Autodesk Fusion 360 part; units mm, degrees
(part 2 of 2)
sketch "스케치2 (4)" plane through (0, 0, 0) normal (0, 0, 1) x (1, 0, 0) in component "right-switch"
  line L0 (143.11, 0) -> (143.11, 105.25)
  line L1 (163.11, 0) -> (338.56, 0)
  line L2 (338.56, 0) -> (338.56, 105.25)
  line L3 (338.56, 105.25) -> (163.11, 105.25)
  line L4 (163.11, 105.25) -> (163.11, 0)
  line L5 (143.11, 105.25) -> (0, 105.25)
  line L6 (322.035, 21.525) -> (336.035, 21.525)
  line L7 (336.035, 21.525) -> (336.035, 7.525)
  line L8 (336.035, 7.525) -> (322.035, 7.525)
  line L9 (322.035, 7.525) -> (322.035, 21.525)
  line L10 (302.985, 21.525) -> (316.985, 21.525)
  line L11 (302.985, 7.525) -> (302.985, 21.525)
  line L12 (316.985, 21.525) -> (316.985, 7.525)
  line L13 (316.985, 7.525) -> (302.985, 7.525)
  line L14 (283.935, 21.525) -> (297.935, 21.525)
  line L15 (283.935, 7.525) -> (283.935, 21.525)
  line L16 (297.935, 21.525) -> (297.935, 7.525)
  line L17 (297.935, 7.525) -> (283.935, 7.525)
  line L18 (264.885, 21.525) -> (278.885, 21.525)
  line L19 (264.885, 7.525) -> (264.885, 21.525)
  line L20 (278.885, 21.525) -> (278.885, 7.525)
  line L21 (278.885, 7.525) -> (264.885, 7.525)
  line L22 (245.835, 21.525) -> (259.835, 21.525)
  line L23 (245.835, 7.525) -> (245.835, 21.525)
  line L24 (259.835, 21.525) -> (259.835, 7.525)
  line L25 (259.835, 7.525) -> (245.835, 7.525)
  line L26 (324.1287, 59.625) -> (324.1287, 53.625)
  line L27 (324.1287, 53.625) -> (325.6287, 53.625)
  line L28 (325.6287, 58.125) -> (332.4287, 58.125)
  line L29 (308.6287, 47.125) -> (301.8287, 47.125)
  line L30 (324.1287, 51.625) -> (324.1287, 45.625)
  line L31 (301.8287, 47.125) -> (301.8287, 58.125)
  line L32 (308.6287, 58.125) -> (308.6287, 53.625)
  line L33 (301.8287, 58.125) -> (308.6287, 58.125)
  line L34 (308.6287, 53.625) -> (310.1287, 53.625)
  line L35 (308.6287, 51.625) -> (308.6287, 47.125)
  line L36 (310.1287, 51.625) -> (308.6287, 51.625)
  line L37 (310.1287, 59.625) -> (324.1287, 59.625)
  line L38 (310.1287, 45.625) -> (310.1287, 51.625)
  line L39 (310.1287, 53.625) -> (310.1287, 59.625)
  line L40 (325.6287, 53.625) -> (325.6287, 58.125)
  line L41 (324.1287, 45.625) -> (310.1287, 45.625)
  line L42 (332.4287, 47.125) -> (325.6287, 47.125)
  line L43 (325.6287, 47.125) -> (325.6287, 51.625)
  line L44 (332.4287, 58.125) -> (332.4287, 47.125)
  line L45 (325.6287, 51.625) -> (324.1287, 51.625)
  line L46 (322.035, 40.575) -> (336.035, 40.575)
  line L47 (336.035, 40.575) -> (336.035, 26.575)
  line L48 (336.035, 26.575) -> (322.035, 26.575)
  line L49 (322.035, 26.575) -> (322.035, 40.575)
  line L50 (312.3662, 26.575) -> (298.3662, 26.575)
  line L51 (312.3662, 40.575) -> (312.3662, 26.575)
  line L52 (298.3663, 40.575) -> (312.3663, 40.575)
  line L53 (298.3663, 26.575) -> (298.3663, 40.575)
  line L54 (288.6975, 26.575) -> (274.6975, 26.575)
  line L55 (288.6975, 40.575) -> (288.6975, 26.575)
  line L56 (274.6975, 40.575) -> (288.6975, 40.575)
  line L57 (274.6975, 26.575) -> (274.6975, 40.575)
  line L58 (255.6475, 40.575) -> (269.6475, 40.575)
  line L59 (255.6475, 26.575) -> (255.6475, 40.575)
  line L60 (269.6475, 40.575) -> (269.6475, 26.575)
  line L61 (269.6475, 26.575) -> (255.6475, 26.575)
  line L62 (236.5975, 40.575) -> (250.5975, 40.575)
  line L63 (236.5975, 26.575) -> (236.5975, 40.575)
  line L64 (250.5975, 40.575) -> (250.5975, 26.575)
  line L65 (250.5975, 26.575) -> (236.5975, 26.575)
  line L66 (217.5475, 40.575) -> (231.5475, 40.575)
  line L67 (217.5475, 26.575) -> (217.5475, 40.575)
  line L68 (231.5475, 40.575) -> (231.5475, 26.575)
  line L69 (231.5475, 26.575) -> (217.5475, 26.575)
  line L70 (198.4975, 40.575) -> (212.4975, 40.575)
  line L71 (198.4975, 26.575) -> (198.4975, 40.575)
  line L72 (212.4975, 40.575) -> (212.4975, 26.575)
  line L73 (212.4975, 26.575) -> (198.4975, 26.575)
  line L74 (179.4475, 40.575) -> (193.4475, 40.575)
  line L75 (179.4475, 26.575) -> (179.4475, 40.575)
  line L76 (193.4475, 40.575) -> (193.4475, 26.575)
  line L77 (193.4475, 26.575) -> (179.4475, 26.575)
  line L78 (193.4475, 7.525) -> (179.4475, 7.525)
  line L79 (193.4475, 21.525) -> (193.4475, 7.525)
  line L80 (179.4475, 7.525) -> (179.4475, 21.525)
  line L81 (179.4475, 21.525) -> (193.4475, 21.525)
  line L82 (212.6412, 15.525) -> (212.6412, 21.525)
  line L83 (228.1412, 15.525) -> (228.1412, 20.025)
  line L84 (228.1412, 9.025) -> (228.1412, 13.525)
  line L85 (204.3412, 20.025) -> (211.1412, 20.025)
  line L86 (204.3412, 9.025) -> (204.3412, 20.025)
  line L87 (228.1412, 20.025) -> (234.9412, 20.025)
  line L88 (226.6412, 7.525) -> (212.6412, 7.525)
  line L89 (211.1412, 15.525) -> (212.6412, 15.525)
  line L90 (211.1412, 9.025) -> (204.3412, 9.025)
  line L91 (212.6412, 13.525) -> (211.1412, 13.525)
  line L92 (211.1412, 20.025) -> (211.1412, 15.525)
  line L93 (211.1412, 13.525) -> (211.1412, 9.025)
  line L94 (226.6412, 13.525) -> (226.6412, 7.525)
  line L95 (234.9412, 20.025) -> (234.9412, 9.025)
  line L96 (212.6412, 21.525) -> (226.6412, 21.525)
  line L97 (226.6412, 21.525) -> (226.6412, 15.525)
  line L98 (226.6412, 15.525) -> (228.1412, 15.525)
  line L99 (212.6412, 7.525) -> (212.6412, 13.525)
  line L100 (234.9412, 9.025) -> (228.1412, 9.025)
  line L101 (228.1412, 13.525) -> (226.6412, 13.525)
  line L102 (281.6975, 45.625) -> (281.6975, 59.625)
  line L103 (295.6975, 59.625) -> (295.6975, 45.625)
  line L104 (281.6975, 59.625) -> (295.6975, 59.625)
  line L105 (295.6975, 45.625) -> (281.6975, 45.625)
  line L106 (262.6475, 59.625) -> (276.6475, 59.625)
  line L107 (276.6475, 59.625) -> (276.6475, 45.625)
  line L108 (276.6475, 45.625) -> (262.6475, 45.625)
  line L109 (262.6475, 45.625) -> (262.6475, 59.625)
  line L110 (243.5975, 59.625) -> (257.5975, 59.625)
  line L111 (257.5975, 59.625) -> (257.5975, 45.625)
  line L112 (257.5975, 45.625) -> (243.5975, 45.625)
  line L113 (243.5975, 45.625) -> (243.5975, 59.625)
  line L114 (224.5475, 59.625) -> (238.5475, 59.625)
  line L115 (238.5475, 59.625) -> (238.5475, 45.625)
  line L116 (238.5475, 45.625) -> (224.5475, 45.625)
  line L117 (224.5475, 45.625) -> (224.5475, 59.625)
  line L118 (205.4975, 59.625) -> (219.4975, 59.625)
  line L119 (219.4975, 59.625) -> (219.4975, 45.625)
  line L120 (219.4975, 45.625) -> (205.4975, 45.625)
  line L121 (205.4975, 45.625) -> (205.4975, 59.625)
  line L122 (186.4475, 59.625) -> (200.4475, 59.625)
  line L123 (200.4475, 59.625) -> (200.4475, 45.625)
  line L124 (200.4475, 45.625) -> (186.4475, 45.625)
  line L125 (186.4475, 45.625) -> (186.4475, 59.625)
  line L126 (331.2725, 64.675) -> (317.2725, 64.675)
  line L127 (317.2725, 78.675) -> (331.2725, 78.675)
  line L128 (317.2725, 64.675) -> (317.2725, 78.675)
  line L129 (331.2725, 78.675) -> (331.2725, 64.675)
  line L130 (309.985, 64.675) -> (295.985, 64.675)
  line L131 (309.985, 78.675) -> (309.985, 64.675)
  line L132 (295.985, 78.675) -> (309.985, 78.675)
  line L133 (295.985, 64.675) -> (295.985, 78.675)
  line L134 (290.935, 78.675) -> (290.935, 64.675)
  line L135 (276.935, 78.675) -> (290.935, 78.675)
  line L136 (290.935, 64.675) -> (276.935, 64.675)
  line L137 (276.935, 64.675) -> (276.935, 78.675)
  line L138 (271.885, 78.675) -> (271.885, 64.675)
  line L139 (257.885, 78.675) -> (271.885, 78.675)
  line L140 (271.885, 64.675) -> (257.885, 64.675)
  line L141 (257.885, 64.675) -> (257.885, 78.675)
  line L142 (252.835, 78.675) -> (252.835, 64.675)
  line L143 (238.835, 78.675) -> (252.835, 78.675)
  line L144 (252.835, 64.675) -> (238.835, 64.675)
  line L145 (238.835, 64.675) -> (238.835, 78.675)
  line L146 (233.785, 78.675) -> (233.785, 64.675)
  line L147 (219.785, 78.675) -> (233.785, 78.675)
  line L148 (233.785, 64.675) -> (219.785, 64.675)
  line L149 (219.785, 64.675) -> (219.785, 78.675)
  line L150 (214.735, 78.675) -> (214.735, 64.675)
  line L151 (200.735, 78.675) -> (214.735, 78.675)
  line L152 (214.735, 64.675) -> (200.735, 64.675)
  line L153 (200.735, 64.675) -> (200.735, 78.675)
  line L154 (195.685, 78.675) -> (195.685, 64.675)
  line L155 (181.685, 78.675) -> (195.685, 78.675)
  line L156 (195.685, 64.675) -> (181.685, 64.675)
  line L157 (181.685, 64.675) -> (181.685, 78.675)
  line L158 (328.01, 85.225) -> (328.01, 89.725)
  line L159 (328.01, 89.725) -> (326.51, 89.725)
  line L160 (312.51, 89.725) -> (311.01, 89.725)
  line L161 (328.01, 91.725) -> (328.01, 96.225)
  line L162 (326.51, 83.725) -> (312.51, 83.725)
  line L163 (312.51, 83.725) -> (312.51, 89.725)
  line L164 (311.01, 96.225) -> (311.01, 91.725)
  line L165 (312.51, 97.725) -> (326.51, 97.725)
  line L166 (326.51, 97.725) -> (326.51, 91.725)
  line L167 (326.51, 91.725) -> (328.01, 91.725)
  line L168 (326.51, 89.725) -> (326.51, 83.725)
  line L169 (304.21, 85.225) -> (304.21, 96.225)
  line L170 (311.01, 91.725) -> (312.51, 91.725)
  line L171 (304.21, 96.225) -> (311.01, 96.225)
  line L172 (334.81, 96.225) -> (334.81, 85.225)
  line L173 (311.01, 89.725) -> (311.01, 85.225)
  line L174 (312.51, 91.725) -> (312.51, 97.725)
  line L175 (334.81, 85.225) -> (328.01, 85.225)
  line L176 (328.01, 96.225) -> (334.81, 96.225)
  line L177 (311.01, 85.225) -> (304.21, 85.225)
  line L178 (286.46, 97.725) -> (300.46, 97.725)
  line L179 (300.46, 97.725) -> (300.46, 83.725)
  line L180 (300.46, 83.725) -> (286.46, 83.725)
  line L181 (286.46, 83.725) -> (286.46, 97.725)
  line L182 (281.41, 83.725) -> (267.41, 83.725)
  line L183 (281.41, 97.725) -> (281.41, 83.725)
  line L184 (267.41, 97.725) -> (281.41, 97.725)
  line L185 (267.41, 83.725) -> (267.41, 97.725)
  line L186 (262.36, 83.725) -> (248.36, 83.725)
  line L187 (262.36, 97.725) -> (262.36, 83.725)
  line L188 (248.36, 97.725) -> (262.36, 97.725)
  line L189 (248.36, 83.725) -> (248.36, 97.725)
  line L190 (243.31, 83.725) -> (229.31, 83.725)
  line L191 (243.31, 97.725) -> (243.31, 83.725)
  line L192 (229.31, 97.725) -> (243.31, 97.725)
  line L193 (229.31, 83.725) -> (229.31, 97.725)
  line L194 (224.26, 83.725) -> (210.26, 83.725)
  line L195 (224.26, 97.725) -> (224.26, 83.725)
  line L196 (210.26, 97.725) -> (224.26, 97.725)
  line L197 (210.26, 83.725) -> (210.26, 97.725)
  line L198 (205.21, 83.725) -> (191.21, 83.725)
  line L199 (205.21, 97.725) -> (205.21, 83.725)
  line L200 (191.21, 97.725) -> (205.21, 97.725)
  line L201 (191.21, 83.725) -> (191.21, 97.725)
  line L202 (186.16, 83.725) -> (172.16, 83.725)
  line L203 (186.16, 97.725) -> (186.16, 83.725)
  line L204 (172.16, 97.725) -> (186.16, 97.725)
  line L205 (172.16, 83.725) -> (172.16, 97.725)
  circle A0 centre (167.11, 101.25) radius 1.55
  circle A1 centre (167.11, 4) radius 1.5
  circle A2 centre (167.11, 4) radius 1.55
  circle A3 centre (266.36, 4) radius 1.55
  circle A4 centre (258.36, 4) radius 1.55
  circle A5 centre (334.56, 4) radius 1.55
  circle A6 centre (334.56, 101.25) radius 1.55
  circle A7 centre (266.36, 101.25) radius 1.55
  circle A8 centre (258.36, 101.25) radius 1.55
  point P0 (143.11, 105.25)
  point P1 (143.11, 0)
  dimension "d237" = 20
  dimension "d238" = 175.45
  dimension "d239" = 14
  dimension "d240" = 14
  dimension "d241" = 7.525
  dimension "d242" = 2.525
  dimension "d246" = 0
  dimension "d251" = 14
  dimension "d252" = 14
  dimension "d253" = 6.8
  dimension "d254" = 11
  dimension "d255" = 1.5
  dimension "d256" = 4.5
  dimension "d257" = 6
  dimension "d261" = 14
  dimension "d262" = 14
  dimension "d263" = 19.05
  dimension "d264" = 2.525
  dimension "d265" = 14
  dimension "d266" = 14
  dimension "d267" = 9.6687
  dimension "d268" = 14
  dimension "d269" = 14
  dimension "d270" = 9.6688
  dimension "d274" = 0
  dimension "d275" = 14
  dimension "d276" = 14
  dimension "d277" = 6.8
  dimension "d278" = 11
  dimension "d279" = 1.5
  dimension "d280" = 4.5
  dimension "d281" = 6
  dimension "d282" = 19.1937
  dimension "d283" = 19.05
  dimension "d284" = 14.4313
  dimension "d285" = 14
  dimension "d286" = 14
  dimension "d287" = 14.4313
  dimension "d291" = 0
  dimension "d292" = 14
  dimension "d293" = 14
  dimension "d294" = 19.05
  dimension "d295" = 7.2875
  dimension "d296" = 14
  dimension "d297" = 14
  dimension "d298" = 7.2875
  dimension "d302" = 0
  dimension "d303" = 14
  dimension "d304" = 14
  dimension "d305" = 6.8
  dimension "d306" = 11
  dimension "d307" = 1.5
  dimension "d308" = 4.5
  dimension "d309" = 6
  dimension "d310" = 19.05
  dimension "d311" = 12.05
  dimension "d312" = 14
  dimension "d313" = 14
  dimension "d314" = 12.05
  dimension "d318" = 0
  dimension "d319" = 3.1
  dimension "d320" = 4
  dimension "d321" = 4
  dimension "d322" = 3
  dimension "d323" = 4
  dimension "d324" = 4
  dimension "d325" = 3.1
  dimension "d326" = 3.1
  dimension "d327" = 72.2
  dimension "d328" = 4
  dimension "d329" = 3.1
  dimension "d330" = 8
  dimension "d331" = 4
  dimension "d332" = 3.1
  dimension "d333" = 4
  dimension "d334" = 4
  dimension "d336" = 3.1
  dimension "d337" = 3.1
  dimension "d338" = 8
  dimension "d339" = 3.1
  dimension "d340" = 4
  dimension "d341" = 4
  constraint vertical L2
  constraint vertical L4
  constraint horizontal L3.end P0
  constraint equal L0 L4
  constraint horizontal L3
  constraint horizontal L1
  constraint horizontal L6
  constraint vertical L7
  constraint horizontal L8
  constraint vertical L9
  constraint horizontal L37
  constraint vertical L26
  constraint horizontal L41
  constraint vertical L38
  constraint horizontal L33
  constraint vertical L32
  constraint horizontal L29
  constraint vertical L31
  constraint horizontal L34
  constraint horizontal L45
  constraint horizontal L28
  constraint vertical L44
  constraint horizontal L42
  constraint vertical L43
  constraint collinear L32 L35
  constraint coincident L36.start L45
  constraint collinear L38 L39
  constraint coincident L26.end L34
  constraint collinear L26 L30
  constraint collinear L40 L43
  constraint collinear L36 L45
  constraint collinear L27 L34
  constraint equal L28 L33
  constraint equal L31 L44
  constraint equal L32 L40
  constraint equal L27 L34
  constraint equal L32 L35
  constraint horizontal L46
  constraint vertical L47
  constraint horizontal L48
  constraint vertical L49
  constraint horizontal L52
  constraint vertical L51
  constraint horizontal L50
  constraint vertical L53
  constraint horizontal L46.start L51.start
  constraint horizontal L56
  constraint vertical L55
  constraint horizontal L54
  constraint vertical L57
  constraint collinear L52 L56
  constraint collinear L75 L80
  constraint collinear L22 L81
  constraint parallel L79 L80
  constraint parallel L78 L81
  constraint equal L77 L81
  constraint equal L23 L79
  constraint horizontal L96
  constraint vertical L97
  constraint horizontal L88
  constraint vertical L99
  constraint horizontal L85
  constraint vertical L92
  constraint horizontal L90
  constraint vertical L86
  constraint horizontal L89
  constraint horizontal L101
  constraint horizontal L87
  constraint vertical L95
  constraint horizontal L100
  constraint vertical L84
  constraint collinear L92 L93
  constraint coincident L91.start L101
  constraint collinear L82 L99
  constraint coincident L97.end L89
  constraint collinear L94 L97
  constraint collinear L83 L84
  constraint collinear L91 L101
  constraint collinear L89 L98
  constraint equal L85 L87
  constraint equal L86 L95
  constraint equal L83 L92
  constraint equal L89 L98
  constraint equal L92 L93
  constraint collinear L22 L96
  constraint coincident L96.end L97.start
  constraint coincident L26.start L37.end
  constraint horizontal L104
  constraint vertical L103
  constraint horizontal L105
  constraint vertical L102
  constraint collinear L37 L104
  constraint horizontal L127
  constraint vertical L129
  constraint horizontal L126
  constraint vertical L128
  constraint horizontal L132
  constraint vertical L131
  constraint horizontal L130
  constraint vertical L133
  constraint collinear L127 L132
  constraint horizontal L165
  constraint vertical L166
  constraint horizontal L162
  constraint vertical L163
  constraint horizontal L171
  constraint vertical L164
  constraint horizontal L177
  constraint vertical L169
  constraint horizontal L170
  constraint horizontal L159
  constraint horizontal L176
  constraint vertical L172
  constraint horizontal L175
  constraint vertical L158
  constraint collinear L164 L173
  constraint coincident L160.start L159
  constraint collinear L163 L174
  constraint coincident L166.end L170
  constraint collinear L166 L168
  constraint collinear L158 L161
  constraint collinear L159 L160
  constraint collinear L167 L170
  constraint equal L171 L176
  constraint equal L169 L172
  constraint equal L161 L164
  constraint equal L167 L170
  constraint equal L164 L173
  constraint coincident L165.end L166.start
  constraint horizontal L178
  constraint vertical L179
  constraint horizontal L180
  constraint vertical L181
  constraint collinear L165 L178
  constraint horizontal A7.centre A6.centre
  constraint vertical A3.centre A7.centre
  constraint horizontal A8.centre A7.centre
  measures "d237" distance of L1.start P1
  measures "d238" distance of L1.start L1.end
  measures "d239" distance of L6.start L6.end
  measures "d240" distance of L6.start L8.end
  measures "d241" vertical distance of L1.end L7.end
  measures "d242" horizontal distance of L1.end L7.end
  measures "d251" distance of L26.start L37.start
  measures "d252" distance of L37.start L38.start
  measures "d253" distance of L31.end L32.start
  measures "d254" distance of L31.end L29.end
  measures "d255" distance of L32.end L34.end
  measures "d256" distance of L32.start L32.end
  measures "d257" distance of L37.start L34.end
  measures "d261" distance of L46.start L46.end
  measures "d262" distance of L46.start L48.end
  measures "d263" distance of L7.end L47.end
  measures "d264" horizontal distance of L1.end L47.end
  measures "d265" distance of L52.start L51.start
  measures "d266" distance of L52.start L53.start
  measures "d267" distance of L48.end L50.start
  measures "d268" distance of L55.start L56.start
  measures "d269" distance of L56.start L54.end
  measures "d270" distance of L53.start L54.start
  measures "d275" distance of L82.end L96.end
  measures "d276" distance of L88.end L82.end
  measures "d277" distance of L85.start L85.end
  measures "d278" distance of L85.start L86.start
  measures "d279" distance of L82.start L89.start
  measures "d280" distance of L85.end L89.start
  measures "d281" distance of L82.end L82.start
  measures "d282" distance of L23.start L88.start
  measures "d283" vertical distance of L26.start L46.end
  measures "d284" distance of L2 L30.end
  measures "d285" distance of L103.start L102.end
  measures "d286" distance of L102.start L102.end
  measures "d287" distance of L38.start L103.end
  measures "d292" distance of L127.start L127.end
  measures "d293" distance of L127.start L126.end
  measures "d294" vertical distance of L26.start L127.end
  measures "d295" distance of L2 L126.start
  measures "d296" distance of L132.start L131.start
  measures "d297" distance of L130.end L132.start
  measures "d298" distance of L126.end L130.start
  measures "d303" distance of L165.start L165.end
  measures "d304" distance of L162.end L165.start
  measures "d305" distance of L169.end L164.start
  measures "d306" distance of L169.end L169.start
  measures "d307" distance of L170.end L164.end
  measures "d308" distance of L164.start L164.end
  measures "d309" distance of L165.start L170.end
  measures "d310" vertical distance of L127.end L165.end
  measures "d311" distance of L2 L162.start
  measures "d312" distance of L178.start L178.end
  measures "d313" distance of L180.end L178.start
  measures "d314" distance of L162.end L179.end
  measures "d319" diameter of A0
  measures "d320" horizontal distance of L3.end A0.centre
  measures "d321" vertical distance of L3.end A0.centre
  measures "d322" diameter of A1
  measures "d323" vertical distance of L1.start A1.centre
  measures "d324" horizontal distance of L1.start A1.centre
  measures "d325" diameter of A2
  measures "d326" diameter of A3
  measures "d327" horizontal distance of L1.end A3.centre
  measures "d328" distance of L1 A3.centre
  measures "d329" diameter of A4
  measures "d330" distance of A3.centre A4.centre
  measures "d331" distance of L1 A4.centre
  measures "d332" diameter of A5
  measures "d333" vertical distance of L1.end A5.centre
  measures "d334" horizontal distance of L1.end A5.centre
  measures "d336" diameter of A7
  measures "d337" diameter of A8
  measures "d338" distance of A8.centre A7.centre
  measures "d339" diameter of A6
  measures "d340" vertical distance of L2.end A6.centre
  measures "d341" horizontal distance of L2.end A6.centre
extrude "돌출1'''" add sketch "스케치2 (4)" along normal blind 3 separate body contours L1 L2 L3 L4 makes body 6 in component "right-switch"
sketch "스케치3" plane through (0, 0, 3) normal (0, 0, 1) x (-1, 0, 0) in component "right-switch"
  circle A0 centre (-167.11, -101.25) radius 1.55
  circle A1 centre (-167.11, -4) radius 1.55
  circle A2 centre (-258.36, -4) radius 1.55
  circle A3 centre (-266.36, -4) radius 1.55
  circle A4 centre (-334.56, -4) radius 1.55
  circle A5 centre (-334.56, -101.25) radius 1.55
  circle A6 centre (-266.36, -101.25) radius 1.55
  circle A7 centre (-258.36, -101.25) radius 1.55
  circle A8 centre (-167.11, -101.25) radius 3
  circle A9 centre (-258.36, -101.25) radius 3
  circle A10 centre (-266.36, -101.25) radius 3
  circle A11 centre (-334.56, -101.25) radius 3
  circle A12 centre (-334.56, -4) radius 3
  circle A13 centre (-266.36, -4) radius 3
  circle A14 centre (-258.36, -4) radius 3
  circle A15 centre (-167.11, -4) radius 3
  dimension "d354" = 6
  dimension "d355" = 6
  dimension "d356" = 6
  dimension "d357" = 6
  dimension "d358" = 6
  dimension "d359" = 6
  dimension "d360" = 6
  dimension "d361" = 6
  constraint concentric A0 A8
  constraint concentric A7 A9
  constraint concentric A6 A10
  constraint concentric A5 A11
  constraint concentric A4 A12
  constraint concentric A3 A13
  constraint concentric A2 A14
  constraint concentric A1 A15
  measures "d354" diameter of A8
  measures "d355" diameter of A9
  measures "d356" diameter of A10
  measures "d357" diameter of A11
  measures "d358" diameter of A12
  measures "d359" diameter of A13
  measures "d360" diameter of A14
  measures "d361" diameter of A15
extrude "돌출2''''" cut sketch "스케치3" against normal blind 1.75 bodies 6 in component "right-switch"
sketch "스케치1 (3)" plane through (0, 0, 0) normal (0, 0, 1) x (1, 0, 0) in component "right-body1"
  line L0 (163.11, 0) -> (338.56, 0)
  line L1 (163.11, 105.25) -> (163.11, 0)
  line L2 (338.56, 105.25) -> (163.11, 105.25)
  circle A0 centre (167.11, 4) radius 1.55
  circle A1 centre (167.11, 101.25) radius 1.55
  circle A2 centre (258.36, 101.25) radius 1.55
  circle A3 centre (258.36, 4) radius 1.55
  circle A4 centre (266.36, 4) radius 1.55
  circle A5 centre (266.36, 101.25) radius 1.55
  line L3 (258.36, 4) -> (266.36, 4) construction
  line L4 (258.36, 101.25) -> (266.36, 101.25) construction
  line L5 (262.36, 4) -> (262.36, 101.25) construction
  line L6 (163.11, 0) -> (167.11, 0)
  line L7 (262.36, 0) -> (262.36, 105.25)
  line L8 (262.36, 105.25) -> (163.11, 105.25)
  line L9 (163.11, 105.25) -> (163.11, 0)
  line L10 (166.11, 7.873) -> (166.11, 97.377)
  line L11 (170.983, 102.25) -> (254.487, 102.25)
  line L12 (254.487, 3) -> (170.983, 3)
  arc A6 (254.487, 102.25) -> (262.36, 101.25) centre (258.36, 101.25) ccw
  arc A7 (166.11, 97.377) -> (170.983, 102.25) centre (167.11, 101.25) ccw
  arc A8 (262.36, 4) -> (254.487, 3) centre (258.36, 4) ccw
  arc A9 (170.983, 3) -> (166.11, 7.873) centre (167.11, 4) ccw
  circle A10 centre (167.11, 4) radius 1.5 construction
  circle A11 centre (258.36, 4) radius 1.5 construction
  circle A12 centre (258.36, 101.25) radius 1.5 construction
  circle A13 centre (167.11, 101.25) radius 1.5 construction
  line L13 (163.11, 0) -> (262.36, 0)
  dimension "d368" = 8
  dimension "d369" = 8
  dimension "d370" = 8
  dimension "d371" = 8
  dimension "d372" = 3
  dimension "d373" = 3
  dimension "d374" = 3
  dimension "d375" = 3
  dimension "d376" = 3
  dimension "d377" = 3
  dimension "d378" = 3
  constraint coincident A3.centre L3.start
  constraint coincident A4.centre L3.end
  constraint coincident A2.centre L4.start
  constraint coincident A5.centre L4.end
  constraint midpoint L3 L5.start
  constraint midpoint L4 L5.end
  constraint horizontal L6
  constraint vertical L7
  constraint horizontal L8
  constraint vertical L9
  constraint coincident L2 L7.end
  constraint coincident L0.start L1.end
  constraint collinear L5 L7
  constraint concentric A0 A9
  constraint concentric A3 A8
  constraint concentric A1 A7
  constraint concentric A2 A6
  constraint vertical L10
  constraint perpendicular L10 L11
  constraint parallel L6 L12
  constraint concentric A9 A10
  constraint concentric A8 A11
  constraint concentric A6 A12
  constraint concentric A7 A13
  constraint horizontal L0.start L7.start
  measures "d368" diameter of A9
  measures "d369" diameter of A8
  measures "d370" diameter of A7
  measures "d371" diameter of A6
  measures "d372" horizontal distance of L0.start L10.start
  measures "d373" vertical distance of L7.start L12.start
  measures "d374" vertical distance of L1.start L11.start
  measures "d375" diameter of A10
  measures "d376" diameter of A11
  measures "d377" diameter of A12
  measures "d378" diameter of A13
extrude "돌출1''''" add sketch "스케치1 (3)" against normal blind 10 separate body contours L0 L1 L2 L6 L7 L8 L9 L10 L11 L12 A6 A7 A8 A9 L13 | L7 L10 L11 L12 A6 A7 A8 A9 | A0 | A1 | A2 | A3 makes body 7 in component "right-body1"
extrude "돌출2'''''" cut sketch "스케치1 (3)" against normal blind 9 contours L7 L10 L11 L12 A6 A7 A8 A9 bodies 7 in component "right-body1"
extrude "돌출3'''" cut sketch "스케치1 (3)" against normal blind 8 contours A0 | A1 | A2 | A3 bodies 7 in component "right-body1"
sketch "스케치1 (4)" plane through (0, 0, 0) normal (0, 0, 1) x (1, 0, 0) in component "right-body2"
  line L0 (338.56, 105.25) -> (163.11, 105.25)
  line L1 (362.61, 105.25) -> (338.56, 105.25)
  line L2 (362.61, 0) -> (362.61, 105.25)
  line L3 (338.56, 0) -> (362.61, 0)
  line L4 (163.11, 0) -> (338.56, 0)
  circle A0 centre (266.36, 4) radius 1.55
  circle A1 centre (334.56, 4) radius 1.55
  circle A2 centre (342.56, 4) radius 1.55
  circle A3 centre (358.61, 4) radius 1.55
  circle A4 centre (266.36, 101.25) radius 1.55
  circle A5 centre (334.56, 101.25) radius 1.55
  circle A6 centre (342.56, 101.25) radius 1.55
  circle A7 centre (358.61, 101.25) radius 1.55
  line L5 (262.36, 4) -> (262.36, 101.25)
  line L6 (362.61, 0) -> (262.36, 0)
  line L7 (262.36, 0) -> (262.36, 105.25)
  line L8 (262.36, 105.25) -> (362.61, 105.25)
  line L9 (362.61, 105.25) -> (362.61, 0)
  line L10 (359.61, 97.377) -> (359.61, 7.873)
  arc A8 (262.36, 101.25) -> (270.233, 102.25) centre (266.36, 101.25) ccw
  arc A9 (330.687, 102.25) -> (338.433, 102.25) centre (334.56, 101.25) ccw
  line L11 (270.233, 102.25) -> (330.687, 102.25)
  arc A10 (338.687, 102.25) -> (346.433, 102.25) centre (342.56, 101.25) ccw
  arc A11 (354.737, 102.25) -> (359.61, 97.377) centre (358.61, 101.25) ccw
  arc A12 (359.61, 7.873) -> (354.737, 3) centre (358.61, 4) ccw
  arc A13 (346.433, 3) -> (338.687, 3) centre (342.56, 4) ccw
  arc A14 (338.433, 3) -> (330.687, 3) centre (334.56, 4) ccw
  line L12 (330.687, 3) -> (270.233, 3)
  line L13 (338.687, 3) -> (338.433, 3)
  line L14 (354.737, 3) -> (346.433, 3)
  arc A15 (270.233, 3) -> (262.36, 4) centre (266.36, 4) ccw
  line L15 (338.433, 102.25) -> (338.687, 102.25)
  line L16 (346.433, 102.25) -> (354.737, 102.25)
  circle A16 centre (266.36, 101.25) radius 1.5
  circle A17 centre (334.56, 101.25) radius 1.5
  circle A18 centre (342.56, 101.25) radius 1.5
  circle A19 centre (358.61, 101.25) radius 1.5
  circle A20 centre (358.61, 4) radius 1.5
  circle A21 centre (342.56, 4) radius 1.5
  circle A22 centre (334.56, 4) radius 1.5
  circle A23 centre (266.36, 4) radius 1.5
  point P0 (266.36, 4)
  point P1 (262.36, 0)
  dimension "d385" = 8
  dimension "d386" = 8
  dimension "d387" = 8
  dimension "d388" = 8
  dimension "d389" = 8
  dimension "d390" = 8
  dimension "d391" = 8
  dimension "d392" = 8
  dimension "d393" = 3
  dimension "d394" = 3
  dimension "d395" = 3
  dimension "d396" = 3
  dimension "d397" = 3
  dimension "d398" = 3
  dimension "d399" = 3
  dimension "d400" = 3
  dimension "d401" = 3
  dimension "d402" = 3
  dimension "d403" = 3
  constraint horizontal L6
  constraint vertical L7
  constraint horizontal L8
  constraint vertical L9
  constraint coincident L2.start L3.end
  constraint collinear L5 L7
  constraint collinear L0 L8
  constraint concentric A4 A8
  constraint concentric A5 A9
  constraint concentric A6 A10
  constraint concentric A7 A11
  constraint concentric A3 A12
  constraint concentric A2 A13
  constraint concentric A1 A14
  constraint coincident P0 A0.centre
  constraint horizontal L11
  constraint perpendicular L10 L11
  constraint perpendicular L10 L14
  constraint coincident A9.end L11
  constraint collinear L11 L15
  constraint coincident A10.end L15
  constraint coincident A13.end L14
  constraint collinear L12 L14
  constraint collinear L13 L14
  constraint collinear L15 L16
  constraint concentric A8 A16
  constraint concentric A9 A17
  constraint concentric A10 A18
  constraint concentric A11 A19
  constraint concentric A12 A20
  constraint concentric A13 A21
  constraint concentric A14 A22
  constraint concentric A15 A23
  measures "d385" diameter of A8
  measures "d386" diameter of A9
  measures "d387" diameter of A10
  measures "d388" diameter of A11
  measures "d389" diameter of A12
  measures "d390" diameter of A13
  measures "d391" diameter of A14
  measures "d392" diameter of A15
  measures "d393" vertical distance of L12.end P1
  measures "d394" horizontal distance of L2.start L10.end
  measures "d395" vertical distance of L1.start A11.start
  measures "d396" diameter of A16
  measures "d397" diameter of A17
  measures "d398" diameter of A18
  measures "d399" diameter of A19
  measures "d400" diameter of A20
  measures "d401" diameter of A21
  measures "d402" diameter of A22
  measures "d403" diameter of A23
extrude "돌출1'''''" add sketch "스케치1 (4)" against normal blind 10 separate body contours A9 A10 L15 | A13 A14 L13 | L0 L1 L2 L3 L4 L6 L7 L8 L9 L10 A8 A9 L11 A10 A11 A12 A13 A14 L12 L14 A15 L16 | L5 L7 L10 A8 A9 L11 A10 A11 A12 A13 A14 L12 L14 A15 L16 | A0 | A1 | A2 | A3 | A4 | A5 | A6 | A7 | A16 | A17 | A18 | A19 | A20 | A21 | A22 | A23 makes body 8 in component "right-body2"
extrude "돌출2''''''" cut sketch "스케치1 (4)" against normal blind 9 contours L5 L7 L10 A8 A9 L11 A10 A11 A12 A13 A14 L12 L14 A15 L16 bodies 8 in component "right-body2"
extrude "돌출3''''" cut sketch "스케치1 (4)" against normal blind 8 contours A0 | A1 | A2 | A3 | A4 | A5 | A6 | A7 | A16 | A17 | A18 | A19 | A20 | A21 | A22 | A23 bodies 8 in component "right-body2"
sketch "스케치2 (5)" plane through (0, 0, -9) normal (0, 0, 1) x (-1, 0, 0) in component "right-body1"
  line L0 (-170.983, -102.25) -> (-254.487, -102.25)
  line L1 (-172.983, -87.25) -> (-184.983, -87.25)
  line L2 (-184.983, -87.25) -> (-184.983, -86.25)
  line L3 (-184.983, -86.25) -> (-172.983, -86.25)
  line L4 (-172.983, -86.25) -> (-172.983, -87.25)
  line L5 (-200.983, -66.65) -> (-218.983, -66.65)
  line L6 (-218.983, -66.65) -> (-218.983, -65.65)
  line L7 (-218.983, -65.65) -> (-200.983, -65.65)
  line L8 (-200.983, -65.65) -> (-200.983, -66.65)
  point P0 (-170.983, -102.25)
  dimension "d410" = 12
  dimension "d411" = 1
  dimension "d412" = 15
  dimension "d413" = 2
  dimension "d414" = 1
  dimension "d415" = 18
  dimension "d416" = 30
  dimension "d417" = 35.6
  constraint horizontal L1
  constraint vertical L2
  constraint horizontal L3
  constraint vertical L4
  constraint horizontal L5
  constraint vertical L6
  constraint horizontal L7
  constraint vertical L8
  measures "d410" distance of L1.start L1.end
  measures "d411" distance of L1.start L3.end
  measures "d412" vertical distance of L1.start P0
  measures "d413" horizontal distance of L1.start P0
  measures "d414" distance of L5.start L7.end
  measures "d415" distance of L6.end L7.end
  measures "d416" horizontal distance of P0 L5.start
  measures "d417" vertical distance of P0 L5.start
extrude "돌출4''" add sketch "스케치2 (5)" along normal blind 2 bodies 7 in component "right-body1"
sketch "스케치4 (2)" plane through (0, 105.25, 0) normal (0, 1, 0) x (-1, 0, 0) in component "right-body1"
  circle A0 centre (-176.383, -6) radius 3.2
  line L0 (-212.883, -7.5) -> (-207.083, -7.5)
  arc A1 (-207.083, -7.5) -> (-207.083, -4.1) centre (-207.083, -5.8) ccw
  line L1 (-207.083, -4.1) -> (-212.883, -4.1)
  arc A2 (-212.883, -4.1) -> (-212.883, -7.5) centre (-212.883, -5.8) ccw
  line L2 (-212.883, -5.8) -> (-207.083, -5.8) construction
  line L3 (-200.983, -9) -> (-218.983, -9)
  line L4 (-212.883, -9.5) -> (-207.083, -9.5)
  arc A3 (-207.083, -9.5) -> (-207.083, -2.1) centre (-207.083, -5.8) ccw
  line L5 (-207.083, -2.1) -> (-212.883, -2.1)
  arc A4 (-212.883, -2.1) -> (-212.883, -9.5) centre (-212.883, -5.8) ccw
  line L6 (-212.883, -5.8) -> (-207.083, -5.8) construction
  point P0 (-170.983, -9)
  dimension "d428" = 6.4
  dimension "d429" = 5.4
  dimension "d430" = 3
  dimension "d433" = 3.4
  dimension "d434" = 5.8
  dimension "d435" = 1.5
  dimension "d436" = 6.1
  dimension "d439" = 3.7
  constraint tangent L0 A1
  constraint tangent A1 L1
  constraint parallel L0 L1
  constraint tangent L1 A2
  constraint tangent L0 A2
  constraint horizontal L2
  constraint tangent L4 A3
  constraint tangent A3 L5
  constraint parallel L4 L5
  constraint tangent L5 A4
  constraint tangent L4 A4
  constraint coincident A1.centre L2.end
  constraint parallel L2 L6
  constraint coincident A2.centre L2.start
  measures "d428" diameter of A0
  measures "d429" horizontal distance of A0.centre P0
  measures "d430" vertical distance of A0.centre P0
  measures "d433" diameter of A1
  measures "d434" distance of L0.start L0.end
  measures "d435" distance of L0.end L3
  measures "d436" horizontal distance of L0.end L3.start
  measures "d439" radius of A3
extrude "돌출7'" cut sketch "스케치4 (2)" against normal blind 2 contours L3 L4 A3 A4 | L3 A3 L5 A4 bodies 7 in component "right-body1"
extrude "돌출6'" cut sketch "스케치4 (2)" against normal blind 3 contours L0 A1 L1 A2 bodies 7 in component "right-body1"
extrude "돌출5'" cut sketch "스케치4 (2)" against normal blind 3 contours A0 bodies 7 in component "right-body1"
sketch "스케치5 (3)" plane through (218.983, 0, 0) normal (1, 0, 0) x (0, 1, 0) in component "right-body1"
  line L0 (65.65, -7) -> (65.65, -6)
  line L1 (65.65, -6) -> (66.977, -7)
  line L2 (66.977, -7) -> (65.65, -7)
  point P0 (65.65, -7)
  dimension "d442" = 1
  dimension "d443" = 37
  constraint vertical L0
  constraint perpendicular L0 L2
  constraint coincident P0 L0.start
  measures "d442" distance of P0 L0.end
  measures "d443" angle of L1 L2
extrude "돌출8" add sketch "스케치5 (3)" against normal blind 18 bodies 7 in component "right-body1"
fillet "모깎기1'" radius 0.2 1 edges at (209.983, 65.65, -6) on bodies 7 in component "right-body1"
fillet "모깎기2" radius 4 2 edges at (163.11, 0, -5) (163.11, 105.25, -5) on bodies 7 in component "right-body1"
fillet "모깎기1''" radius 4 2 edges at (362.61, 105.25, -5) (362.61, 0, -5) on bodies 8 in component "right-body2"
fillet "모깎기1'''" radius 4 2 edges at (163.11, 0, 1.5) (163.11, 105.25, 1.5) on bodies 6 in component "right-switch"
fillet "모깎기1''''" radius 4 2 edges at (-24.05, 105.25, 1.5) (-24.05, 0, 1.5) on bodies 3 in component "right-side-switch"
fillet "모깎기1'''''" radius 4 2 edges at (143.11, 0, 1.5) (143.11, 105.25, 1.5) on bodies 2 in component "left-switch"
fillet "모깎기1''''''" radius 4 2 edges at (-24.05, 105.25, -5) (-24.05, 0, -5) on bodies 4 in component "left-body1"
fillet "모깎기2'" radius 4 2 edges at (143.11, 105.25, -5) (143.11, 0, -5) on bodies 5 in component "left-body2"
component "right-side-switch" placed x (1, 0, 0) y (0, 1, 0) z (0, 0, 1) at (0, 0, 0)
component "left-switch" placed x (1, 0, 0) y (0, 1, 0) z (0, 0, 1) at (0, 0, 0)
component "left-body1" placed x (1, 0, 0) y (0, 1, 0) z (0, 0, 1) at (0, 0, 0)
component "left-body2" placed x (1, 0, 0) y (0, 1, 0) z (0, 0, 1) at (0, 0, 0)
component "right-switch" placed x (1, 0, 0) y (0, 1, 0) z (0, 0, 1) at (0, 0, 0)
component "right-side-switch" placed x (-1, 0, 0) y (0, -1, 0) z (0, 0, 1) at (338.56, 105.25, 0)
component "right-body1" placed x (1, 0, 0) y (0, 1, 0) z (0, 0, 1) at (0, 0, 0)
component "right-body2" placed x (1, 0, 0) y (0, 1, 0) z (0, 0, 1) at (0, 0, 0)
equation "d10 = width"
equation "d11 = width"
equation "d14 = ( ( 19.05 - 14 ) / 2 ) * 1 mm"
equation "d15 = d14"
equation "d20 = width"
equation "d21 = width"
equation "d22 = d14"
equation "d23 = ( space * 1.5 - width ) / 2"
equation "d36 = width"
equation "d37 = width"
equation "d38 = d23 + margin"
equation "width = 14 mm"
equation "space = 19.05 mm"
equation "margin = ( space - width ) / 2"
equation "d44 = space"
equation "d46 = width"
equation "d47 = width"
equation "d48 = ( ( 19.04 * 1.75 - 14 ) / 2 ) * 1 mm"
equation "d49 = margin"
equation "d50 = width"
equation "d51 = width"
equation "d52 = d48 + margin"
equation "d55 = space"
equation "d57 = width"
equation "d58 = width"
equation "d59 = margin"
equation "d60 = ( space * 2.25 - 14 mm ) / 2"
equation "d61 = width"
equation "d62 = width"
equation "d63 = d60 + margin"
equation "d66 = space"
equation "d68 = width"
equation "d69 = width"
equation "d70 = ( space * 1.25 - width ) / 2"
equation "d71 = margin"
equation "d74 = space * 1.25"
equation "d82 = width"
equation "d83 = width"
equation "d89 = ( 1.25 * space - 14 mm ) / 2 + ( 2.25 * space - 14 mm ) / 2"
equation "d90 = bHole1"
equation "d94 = bHole1"
equation "d97 = bHole1"
equation "d100 = bHole1"
equation "d103 = bHole1"
equation "d105 = bHole1"
equation "d107 = bHole1"
equation "d110 = bHole1"
equation "d127 = space + 5 mm"
equation "d128 = width"
equation "d129 = width"
equation "d130 = ( space - 14 mm ) / 2"
equation "d131 = 5 mm + margin"
equation "d135 = space"
equation "d139 = bHole1"
equation "d142 = bHole1"
equation "d145 = bHole1"
equation "d146 = bHole1"
equation "d208 = ( 3.7 * 2 ) * 1 mm"
equation "d239 = width"
equation "d240 = width"
equation "d241 = margin + 5 mm"
equation "d242 = margin"
equation "d245 = -space"
equation "d251 = width"
equation "d252 = width"
equation "d261 = width"
equation "d262 = width"
equation "d264 = margin"
equation "d265 = width"
equation "d266 = width"
equation "d267 = ( ( 19.05 * 1.75 - 14 ) / 2 ) * 1 mm"
equation "d268 = width"
equation "d269 = width"
equation "d270 = ( 1.75 * space - 14 mm ) / 2"
equation "d273 = -space"
equation "d275 = width"
equation "d276 = width"
equation "d282 = ( 2.75 * space - width ) / 2"
equation "d283 = space"
equation "d284 = ( 2.25 * space - 14 mm ) / 2"
equation "d285 = width"
equation "d286 = width"
equation "d287 = ( 2.25 * space - width ) / 2"
equation "d290 = -space"
equation "d292 = width"
equation "d293 = width"
equation "d294 = space"
equation "d295 = ( 1.5 * space - width ) / 2"
equation "d296 = width"
equation "d297 = width"
equation "d298 = ( 1.5 * space - width ) / 2"
equation "d301 = -space"
equation "d303 = width"
equation "d304 = width"
equation "d310 = space"
equation "d311 = ( space * 2 - width ) / 2"
equation "d312 = width"
equation "d313 = width"
equation "d314 = ( 2 * space - width ) / 2"
equation "d317 = -space"
equation "d319 = bHole1"
equation "d325 = bHole1"
equation "d326 = bHole1"
equation "d329 = bHole1"
equation "d332 = bHole1"
equation "d336 = bHole1"
equation "d337 = bHole1"
equation "d339 = bHole1"
equation "d436 = ( ( 18 - 5.8 ) / 2 ) * 1 mm"
equation "d439 = ( 7.4 / 2 ) * 1 mm"
equation "bHole1 = 3.1 mm"
named bodies: "left-switch"
